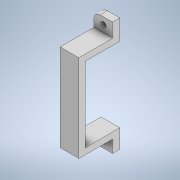
# Autodesk Inventor part: holder servo
Saved by Autodesk Inventor 2020 (Build 240168000, 168)
## iProperties
Created: 2026-07-08
Part Number: holder servo
Material: Generic
Document SubType Name: Modeling
Designer: drago
Density: 1 g/cm^3
Appearance: Default
Author: drago
Autodesk Inventor part; units mm, degrees
ref_plane "YZ Plane" through (0, 0, 0) normal (1, 0, 0) x (0, 1, 0)
ref_plane "XZ Plane" through (0, 0, 0) normal (0, 1, 0) x (-1, 0, 0)
ref_plane "XY Plane" through (0, 0, 0) normal (0, 0, 1) x (1, 0, 0)
sketch "Sketch1" plane through (0, 0, 0) normal (0, 0, 1) x (1, 0, 0)
  line L0 (-7, -17) -> (7, -17)
  line L1 (-7, -17) -> (-1, -17)
  line L2 (-1, -17) -> (-1, -11)
  line L3 (-1, -11) -> (-7, -11)
  line L4 (-7, -11) -> (-7, -17)
  line L5 (-5, 19.5) -> (-0.9, 19.5)
  line L6 (-0.9, 19.5) -> (-0.9, 13)
  line L7 (-0.9, 13) -> (-7, 13)
  line L8 (-7, 13) -> (-7, 17.5)
  line L9 (-7, 17.5) -> (-7, -20)
  line L10 (-0.9, 13) -> (-7, 13)
  line L11 (-7, 13) -> (-7, 15)
  line L12 (-7, 15) -> (-0.9, 15)
  line L13 (-0.9, 15) -> (-0.9, 13)
  line L14 (-7, -11) -> (-1, -11)
  line L15 (-1, -11) -> (-1, -13)
  line L16 (-1, -13) -> (-7, -13)
  line L17 (-7, -13) -> (-7, -11)
  circle A0 centre (-3.95, 17.25) radius 0.9
  circle A1 centre (-4, -15) radius 0.9
  arc A2 (-5, 19.5) -> (-7, 17.5) centre (-5, 17.5) ccw
  point P0 (0, 0)
  point P1 (0, 0)
  point P2 (-0.9, 15)
  dimension "d0" = 2
  constraints: 36 end point, 8 parallel, 4 horizontal, 4 perpendicular, 4 point on circle, 3 centre point, 2 point on line
  measures "d0" distance of L14.end L16.start
extrude "Extrusion1" add sketch "Sketch1" along normal blind 3 contours L4 L16 L2 L0 | L8 A2 L5 L6 L12
extrude "Extrusion2" add sketch "Sketch1" along normal blind 11.8 contours L8 L12 L6 L7 | L4 L3 L2 L16
sketch "Sketch2" plane through (0, 0, 11.8) normal (0, 0, 1) x (1, 0, 0)
  line L0 (-7, 15) -> (-0.9, 15) projected
  line L1 (-1, -13) -> (-7, -13) projected
  line L2 (-0.9, 15) -> (-7, 15)
  line L3 (-7, 15) -> (-7, -13)
  line L4 (-7, -13) -> (-0.9, -13)
  line L5 (-0.9, -13) -> (-0.9, 15)
  point P0 (0, 0)
  constraints: 8 end point, 2 parallel, 1 horizontal, 1 perpendicular
extrude "Extrusion3" add sketch "Sketch2" along normal blind 2
sketch "Sketch3" plane through (-0.9, 19.5, 3) normal (1, 0, 0) x (0, 0, -1)
  line L0 (3, -6.5) -> (3, 0) projected
  line L1 (3, 0) -> (0, 0) projected
  line L2 (0, -4.5) -> (0, 0) projected
  line L3 (0, -4.5) -> (-10.8, -4.5) projected
  line L4 (-10.8, -32.5) -> (-10.8, -4.5) projected
  line L5 (-8.8, -32.5) -> (-10.8, -32.5) projected
  line L6 (-8.8, -32.5) -> (-8.8, -6.5) projected
  line L7 (3, -6.5) -> (-8.8, -6.5) projected
  point P0 (3, -19.5)
extrude "Extrusion4" cut sketch "Sketch3" against normal up to surface (0.1 mm away)
sketch "Sketch4" plane through (0, 0, 0) normal (0, 0, -1) x (-1, 0, 0)
  line L0 (12.228, 25.7128) -> (-5.2106, 25.7128)
  line L1 (-5.2106, 25.7128) -> (-5.2106, -24.037)
  line L2 (-5.2106, -24.037) -> (12.228, -24.037)
  line L3 (12.228, -24.037) -> (12.228, 25.7128)
  point P0 (0, 0)
  constraints: 8 end point, 2 parallel, 1 horizontal, 1 perpendicular
extrude "Extrusion5" cut sketch "Sketch4" against normal blind 0.7
body "Solid1"
